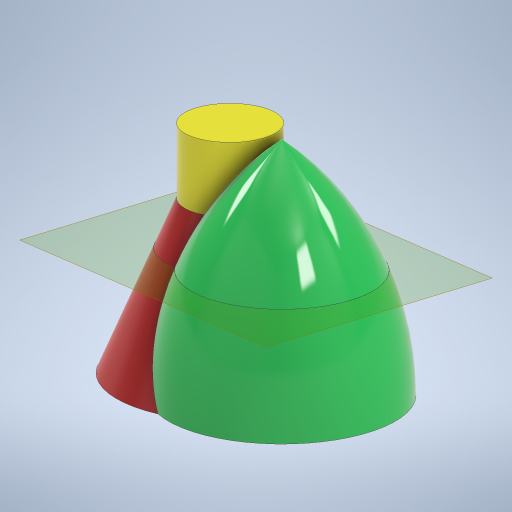
# Autodesk Inventor part: Пример1
Saved by Autodesk Inventor 2023.2 (Build 272271030, 271C)
## iProperties
Created: 2024-10-19
Part Number: Пример1
Material: Типовые
Document SubType Name: Modeling
Designer: stud517
Density: 1 g/cm^3
Appearance: По умолчанию
Author: stud517
Autodesk Inventor part; units mm, degrees
ref_plane "YZ Plane" through (0, 0, 0) normal (1, 0, 0) x (0, 1, 0)
ref_plane "XZ Plane" through (0, 0, 0) normal (0, 1, 0) x (-1, 0, 0)
ref_plane "XY Plane" through (0, 0, 0) normal (0, 0, 1) x (1, 0, 0)
sketch "Эскиз1" plane through (0, 0, 0) normal (0, 0, 1) x (1, 0, 0)
  line L0 (0, 0) -> (50, 0)
  line L1 (0, 0) -> (0, 100)
  line L2 (0, 100) -> (20, 100)
  line L3 (20, 100) -> (20, 70)
  line L4 (20, 70) -> (50, 0)
  dimension "d0" = 50
  dimension "d1" = 100
  dimension "d2" = 20
  dimension "d3" = 30
  constraints: 10 end point, 2 horizontal, 1 perpendicular, 1 vertical
  measures "d0" distance of L0.start L0.end
  measures "d1" distance of L0.start L1.end
  measures "d2" distance of L1.end L2.end
  measures "d3" distance of L2.end L3.end
revolve "Вращение1" add sketch "Эскиз1" angle 360 about axis through (0, 0, 0) along (0, 1, 0)
sketch "Эскиз2" plane through (0, 0, 0) normal (0, 0, 1) x (1, 0, 0)
  line L0 (50, 0) -> (-50, 0) projected
  line L1 (30, 0) -> (80, 0)
  arc A0 (80, 0) -> (30, 102.4695) centre (-50, 0) ccw
  line L2 (30, 0) -> (30, 102.4695)
  point P0 (0, 0)
  dimension "d6" = 50
  constraints: 4 end point, 2 point on circle, 1 centre point, 1 coincident, 1 point on line, 1 vertical
  measures "d6" distance of L1.start L1.end
revolve "Вращение2" add sketch "Эскиз2" angle 360 about axis through (30, 0, 0) along (0, 1, 0)
sketch "Эскиз3" plane through (0, 0, 0) normal (0, 1, 0) x (-1, 0, 0)
  point P0 (0, 0)
ref_plane "РабПлоскость1" through (0, 50, 0) normal (0, -1, 0) x (1, 0, 0)
split body "Разделение1" result two bodies by plane through (0, 50, 0) normal (0, -1, 0) first body at (35.2447, 0.5, -10.7096)
